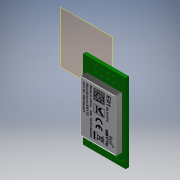
# Autodesk Inventor part: E01-ML01DP5
Saved by Autodesk Inventor 2019 (Build 230136000, 136)
## iProperties
Created: 2019-10-02
Part Number: E01-ML01DP5
Material: Generic
Document SubType Name: Modeling
Designer: rybit
Density: 1 g/cm^3
Appearance: E01-ML01DP5, E01-ML01DP5
Author: rybit
Autodesk Inventor part; units mm, degrees
ref_plane "YZ Plane" through (0, 0, 0) normal (1, 0, 0) x (0, 1, 0)
ref_plane "XZ Plane" through (0, 0, 0) normal (0, 1, 0) x (-1, 0, 0)
ref_plane "XY Plane" through (0, 0, 0) normal (0, 0, 1) x (1, 0, 0)
ref_plane "Work Plane1" through (0, 0, 1) normal (0, 0, 1) x (1, 0, 0)
sketch "Sketch2" plane through (0, 0, 1) normal (0, 0, 1) x (1, 0, 0)
  circle A0 centre (-25.527, 21.082) radius 1.5875 projected
  circle A1 centre (-25.527, -29.718) radius 1.5875 projected
  circle A2 centre (21.463, 21.082) radius 1.5875 projected
  circle A3 centre (21.463, -29.718) radius 1.5875 projected
  circle A4 centre (20.213, 14.652) radius 0.595 projected
  circle A5 centre (20.213, 9.652) radius 0.595 projected
  circle A6 centre (20.213, 4.652) radius 0.595 projected
  circle A7 centre (-25.527, 4.572) radius 0.51 projected
  circle A8 centre (-25.527, 2.032) radius 0.51 projected
  circle A9 centre (-25.527, -0.508) radius 0.51 projected
  circle A10 centre (-25.527, -9.398) radius 0.51 projected
  circle A11 centre (-25.527, -6.858) radius 0.51 projected
  circle A12 centre (7.493, 13.462) radius 0.5 projected
  circle A13 centre (10.033, 13.462) radius 0.5 projected
  circle A14 centre (12.573, 13.462) radius 0.5 projected
  circle A15 centre (12.773, -3.988) radius 0.5 projected
  circle A16 centre (7.693, -1.448) radius 0.5 projected
  circle A17 centre (16.273, -30.798) radius 0.5 projected
  circle A18 centre (13.733, -30.798) radius 0.5 projected
  circle A19 centre (4.273, -30.798) radius 0.5 projected
  circle A20 centre (1.733, -30.798) radius 0.5 projected
  circle A21 centre (7.693, -3.988) radius 0.5 projected
  circle A22 centre (5.153, -1.448) radius 0.5 projected
  circle A23 centre (5.153, -3.988) radius 0.5 projected
  circle A24 centre (12.773, -1.448) radius 0.5 projected
  circle A25 centre (10.233, -3.988) radius 0.5 projected
  circle A26 centre (10.233, -1.448) radius 0.5 projected
  circle A27 centre (-19.427, 6.092) radius 0.5 projected
  circle A28 centre (-19.427, 3.552) radius 0.5 projected
  circle A29 centre (-19.427, 1.012) radius 0.5 projected
  circle A30 centre (-19.427, -1.528) radius 0.5 projected
  circle A31 centre (-19.427, -4.068) radius 0.5 projected
  circle A32 centre (-19.427, -6.608) radius 0.5 projected
  circle A33 centre (-19.427, -9.148) radius 0.5 projected
  circle A34 centre (-19.427, -11.688) radius 0.5 projected
  circle A35 centre (-19.427, -14.228) radius 0.5 projected
  circle A36 centre (-19.427, -16.768) radius 0.5 projected
  circle A37 centre (-19.427, -19.308) radius 0.5 projected
  circle A38 centre (-19.427, -21.848) radius 0.5 projected
  circle A39 centre (-19.427, -24.388) radius 0.5 projected
  circle A40 centre (-19.427, -26.928) radius 0.5 projected
  circle A41 centre (-19.427, -29.468) radius 0.5 projected
  circle A42 centre (-4.187, 6.092) radius 0.5 projected
  circle A43 centre (-4.187, 3.552) radius 0.5 projected
  circle A44 centre (-4.187, 1.012) radius 0.5 projected
  circle A45 centre (-4.187, -1.528) radius 0.5 projected
  circle A46 centre (-4.187, -4.068) radius 0.5 projected
  circle A47 centre (-4.187, -6.608) radius 0.5 projected
  circle A48 centre (-4.187, -9.148) radius 0.5 projected
  circle A49 centre (-4.187, -11.688) radius 0.5 projected
  circle A50 centre (-4.187, -14.228) radius 0.5 projected
  circle A51 centre (-4.187, -16.768) radius 0.5 projected
  circle A52 centre (-4.187, -19.308) radius 0.5 projected
  circle A53 centre (-4.187, -21.848) radius 0.5 projected
  circle A54 centre (-4.187, -24.388) radius 0.5 projected
  circle A55 centre (-4.187, -26.928) radius 0.5 projected
  circle A56 centre (-4.187, -29.468) radius 0.5 projected
  circle A57 centre (0.893, 13.462) radius 0.405 projected
  circle A58 centre (3.433, 13.462) radius 0.405 projected
  circle A59 centre (1.143, 5.842) radius 0.405 projected
  circle A60 centre (3.683, 5.842) radius 0.405 projected
  circle A61 centre (9.143, 21.672) radius 0.4 projected
  circle A62 centre (10.413, 19.732) radius 0.4 projected
  circle A63 centre (11.933, 21.672) radius 0.4 projected
  circle A64 centre (13.463, 19.732) radius 0.4 projected
  circle A65 centre (-24.257, -23.368) radius 0.375 projected
  circle A66 centre (-24.257, -20.828) radius 0.375 projected
  circle A67 centre (-24.257, -18.288) radius 0.375 projected
  circle A68 centre (-25.527, 9.942) radius 0.35 projected
  circle A69 centre (-25.527, 11.442) radius 0.35 projected
  circle A70 centre (-25.527, 12.942) radius 0.35 projected
  circle A71 centre (-25.527, 14.442) radius 0.35 projected
  circle A72 centre (-16.002, 5.842) radius 0.254 projected
  circle A73 centre (-3.302, 7.747) radius 0.254 projected
  circle A74 centre (-12.192, 4.572) radius 0.254 projected
  circle A75 centre (-5.842, -1.778) radius 0.254 projected
  circle A76 centre (-12.192, -3.683) radius 0.254 projected
  circle A77 centre (-19.812, 9.017) radius 0.254 projected
  circle A78 centre (-22.352, -11.303) radius 0.254 projected
  circle A79 centre (-21.717, -7.493) radius 0.254 projected
  circle A80 centre (-10.922, -12.573) radius 0.254 projected
  circle A81 centre (-10.922, 7.112) radius 0.254 projected
  circle A82 centre (-9.652, -11.303) radius 0.254 projected
  circle A83 centre (-7.112, 9.017) radius 0.254 projected
  line L0 (25.273, 24.892) -> (-29.337, 24.892) projected
  line L1 (-29.337, 24.892) -> (-29.337, -33.528) projected
  line L2 (-29.337, -33.528) -> (25.273, -33.528) projected
  line L3 (25.273, -33.528) -> (25.273, 24.892) projected
  line L4 (18, -43) -> (18, 0.1016) projected
  line L5 (-0.1016, 0.1016) -> (-0.1016, -43) projected
  line L6 (18, 0.1016) -> (-0.1016, 0.1016)
  line L7 (-0.1016, 0.1016) -> (-0.1016, -33.3629)
  line L8 (-0.1016, -33.3629) -> (18, -33.3629)
  line L9 (18, -33.3629) -> (18, 0.1016)
  point P0 (0, 0)
  dimension "d3" = 33.4645
  constraints: 8 end point, 2 parallel, 1 horizontal, 1 perpendicular, 1 point on line
  measures "d3" distance between parallel lines of L8 L6
extrude "Extrusion2" add sketch "Sketch2" along normal blind 1.3716 contours L8 L5 L6 L4
sketch "Sketch3" plane through (0, 0, 2.3716) normal (0, 0, 1) x (1, 0, 0)
  circle A0 centre (10.233, -1.448) radius 0.5 projected
  circle A1 centre (10.233, -3.988) radius 0.5 projected
  circle A2 centre (12.773, -1.448) radius 0.5 projected
  circle A3 centre (5.153, -3.988) radius 0.5 projected
  circle A4 centre (5.153, -1.448) radius 0.5 projected
  circle A5 centre (7.693, -3.988) radius 0.5 projected
  circle A6 centre (1.733, -30.798) radius 0.5 projected
  circle A7 centre (4.273, -30.798) radius 0.5 projected
  circle A8 centre (13.733, -30.798) radius 0.5 projected
  circle A9 centre (16.273, -30.798) radius 0.5 projected
  circle A10 centre (7.693, -1.448) radius 0.5 projected
  circle A11 centre (12.773, -3.988) radius 0.5 projected
  line L0 (18, 0.1016) -> (-0.1016, 0.1016) projected
  line L1 (-0.1016, 0.1016) -> (-0.1016, -33.3629) projected
  line L2 (-0.1016, -33.3629) -> (18, -33.3629) projected
  line L3 (18, -33.3629) -> (18, 0.1016) projected
  line L4 (16.476, -28.0924) -> (1.4265, -28.0924)
  line L5 (1.4265, -28.0924) -> (1.4265, -6.0198)
  line L6 (1.4265, -6.0198) -> (16.476, -6.0198)
  line L7 (16.476, -6.0198) -> (16.476, -28.0924)
  point P0 (0, 0)
  dimension "d6" = 15.0495
  dimension "d7" = 22.0726
  dimension "d8" = 5.2705
  dimension "d9" = 1.524
  constraints: 8 end point, 2 parallel, 1 horizontal, 1 perpendicular
  measures "d6" distance of L4.start L4.end
  measures "d7" distance of L4.end L5.end
  measures "d8" distance between parallel lines of L2 L4
  measures "d9" distance between parallel lines of L3 L7
extrude "Extrusion3" add sketch "Sketch3" along normal blind 2.6543 contours L4 L5 L6 L7
fillet "Fillet1" radius 0.2286 8 edges at (16.476, -17.0561, 5.0259) (8.9513, -6.0198, 5.0259) (1.4265, -17.0561, 5.0259) (8.9513, -28.0924, 5.0259) (16.476, -28.0924, 3.6988) (1.4265, -28.0924, 3.6988) (16.476, -6.0198, 3.6988) (1.4265, -6.0198, 3.6988)
sketch "Sketch4" plane through (0, 0, 5.0259) normal (0, 0, 1) x (1, 0, 0)
  line L0 (16.2703, -6.3451) -> (16.2703, -27.5869) construction
  line L1 (16.2703, -27.5869) -> (1.6519, -27.5869) construction
  line L2 (1.6519, -27.5869) -> (1.6519, -6.3451) construction
  line L3 (1.6519, -6.3451) -> (16.2703, -6.3451) construction
  point P0 (0, 0)
  constraints: 2 other
decal "Decal1"
body "Solid1"
